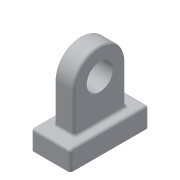
# Autodesk Inventor part: Part1
Saved by Autodesk Inventor 2014 (Build 180170000, 170)
## iProperties
Created: 2013-07-16
Part Number: Part1
Material: Generic
Document SubType Name: Modeling
Density: 1 g/cm^3
Appearance: Default
Autodesk Inventor part; units mm, degrees
ref_plane "YZ Plane" through (0, 0, 0) normal (1, 0, 0) x (0, 1, 0)
ref_plane "XZ Plane" through (0, 0, 0) normal (0, 1, 0) x (-1, 0, 0)
ref_plane "XY Plane" through (0, 0, 0) normal (0, 0, 1) x (1, 0, 0)
sketch "Sketch1" plane through (0, 0, 0) normal (0, 0, 1) x (1, 0, 0)
  line L0 (-15, 30) -> (15, 30)
  line L1 (15, 30) -> (15, -30)
  line L2 (15, -30) -> (-15, -30)
  line L3 (-15, -30) -> (-15, 30)
  line L4 (-15, 30) -> (15, -30) construction
  line L5 (15, 30) -> (-15, -30) construction
  point P0 (0, 0)
  dimension "d0" = 30
  dimension "d1" = 60
  constraints: 12 end point, 2 midpoint, 2 parallel, 1 horizontal, 1 perpendicular
  measures "d0" distance of L1.end L2.end
  measures "d1" distance of L0.end L1.end
extrude "Extrusion1" add sketch "Sketch1" along normal blind 15
sketch "Sketch3" plane through (0, 0, 0) normal (1, 0, 0) x (0, 1, 0)
  line L0 (-20, 15) -> (-20, 45)
  arc A0 (20, 45) -> (-20, 45) centre (0, 45) ccw
  line L1 (20, 45) -> (20, 15)
  line L2 (20, 15) -> (-20, 15)
  line L3 (-30, 15) -> (30, 15) projected
  line L4 (-30, 0) -> (-30, 15) projected
  circle A1 centre (0, 45) radius 10
  point P0 (0, 0)
  dimension "d10" = 30
  dimension "d11" = 20
  dimension "d12" = 10
  dimension "d13" = 20
  constraints: 6 end point, 2 centre point, 2 point on circle, 2 tangent, 1 coincident, 1 collinear, 1 parallel, 1 perpendicular, 1 vertical
  measures "d10" distance of L0.start L0.end
  measures "d11" radius of A0
  measures "d12" distance between parallel lines of L0 L4
  measures "d13" diameter of A1
extrude "Extrusion3" add sketch "Sketch3" along normal mid plane 15
fillet "Fillet1" radius 2 10 edges at (7.5, 0, 65) (7.5, 20, 30) (7.5, -20, 30) (-7.5, 20, 30) (-7.5, -20, 30) (-7.5, 0, 65) (0, -20, 15) (7.5, 0, 15) (0, 20, 15) (-7.5, 0, 15)
fillet "Fillet2" radius 2 8 edges at (15, 0, 15) (0, 30, 15) (-15, 0, 15) (0, -30, 15) (-15, 30, 7.5) (-15, -30, 7.5) (15, 30, 7.5) (15, -30, 7.5)
body "Solid1"
